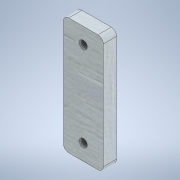
# Autodesk Inventor part: ramie 03-3
Saved by Autodesk Inventor 2021 (Build 250183000, 183)
## iProperties
Created: 2021-11-05
Part Number: ramie 03-3
Material: Generic
Document SubType Name: Modeling
Designer: Łukasz
Density: 1 g/cm^3
Appearance: Wood - Painted White
Author: Łukasz
Autodesk Inventor part; units mm, degrees
ref_plane "YZ Plane" through (0, 0, 0) normal (1, 0, 0) x (0, 1, 0)
ref_plane "XZ Plane" through (0, 0, 0) normal (0, 1, 0) x (-1, 0, 0)
ref_plane "XY Plane" through (0, 0, 0) normal (0, 0, 1) x (1, 0, 0)
sketch "Sketch1" plane through (0, 0, 0) normal (0, 0, 1) x (1, 0, 0)
  arc A0 (2, 32) -> (0, 30) centre (2, 30) ccw
  line L0 (0, 30) -> (0, 20)
  line L1 (15, 20) -> (0, 20)
  line L2 (15, 30) -> (15, 20)
  arc A1 (15, 30) -> (13, 32) centre (13, 30) ccw
  line L3 (13, 32) -> (2, 32)
  arc A2 (0, -10) -> (2, -12) centre (2, -10) ccw
  line L4 (13, -12) -> (2, -12)
  arc A3 (13, -12) -> (15, -10) centre (13, -10) ccw
  line L5 (15, -10) -> (15, 0)
  line L6 (15, 0) -> (0, 0)
  line L7 (0, -10) -> (0, 0)
  line L8 (15, 20) -> (15, 0)
  line L9 (0, 20) -> (0, 0)
  point P0 (15, 24)
  constraints: 20 end point, 8 point on circle, 4 centre point, 2 collinear
extrude "Extrusion1" add sketch "Sketch1" along normal blind 5
sketch "Sketch2" plane through (0, 0, 5) normal (0, 0, 1) x (1, 0, 0)
  circle A0 centre (7.5, -6) radius 1.5
  line L0 (15, -10) -> (15, 30) projected
  circle A1 centre (7.5, 26) radius 1.5
  point P0 (0, 0)
  dimension "d2" = 3
  dimension "d3" = 7.5
  dimension "d4" = 3
  constraints: 2 centre point
  measures "d2" diameter of A0
  measures "d3" distance from line of L0 A0.centre
  measures "d4" diameter of A1
extrude "Extrusion2" cut sketch "Sketch2" against normal up to surface (5 mm away)
body "Solid1"
